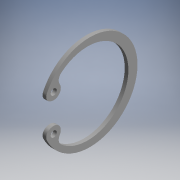
# Autodesk Inventor part: RRING-C-INT-S-30
Saved by Autodesk Inventor 2017.3 (Build 213256000, 256)
## iProperties
Part Number: RRING-C-INT-S-30
Material: Generic
Catalog Web Link: www.cadenas.de
Description: RRING_C_INT-Retaining Rings - C  (Internal)
Vendor: MISUMI
Document SubType Name: Modeling
Designer: partserver
Manufacturer: MISUMI
Mass: 0.253021 g
Surface Area: 6.4299 cm^2
Volume: 0.253021 cm^3
Density: 1 g/cm^3
Appearance: PSOLRGB-192-192-192
Category: PARTsolutions
Company: MISUMI
Title: RRING-C-INT-S-30
Author: Cadenas PARTsolutions
Comments: Retaining Rings - C  (Internal)
PSOL_IDENT_0: {$CADENAS_DATA\23d-libs\misumi\metric\accessories\rring_c_int.prj},181 {VTYP=3D},{NB=RRING-C-INT-S-3
PSOL_IDENT_1: 0},{LINA=RRING-C-INT-S-30},{NN=RRING_C_INT},{DATE=30.10.2020 15:47:10},{GEOMDATE=05.03.2015 00:00:00
PSOL_IDENT_2: },{VERSION=},{LINEID=160},{WBVAR=MAT},{WBNUMERIC=}  {NB=RRING-C-INT-S-30},{LINA=RRING-C-INT-S-30},{K
PSOL_IDENT_3: T=DUMMY},{PN=RRING-C-INT-S-30},{TYPE=RRING-C-INT},{MAT=-S},{HARD=36~44HRC},{NO=30},{DD3=32.1},{DD3TO
PSOL_IDENT_4: L=+0.25/-0.25},{TT=1.20},{TTTOL=+0.06/-0.06},{BB=3.0},{AA=4.7},{DD0=2.0},{DD4=20},{DD1=30},{DD2=31.4
PSOL_IDENT_5: },{DD2TOL=+0.25/0},{MM=1.35},{MMTOL=+0.14/0},{NN=1.5},{A2=12.00}
NB: RRING-C-INT-S-30
NN: 1.5
NT: Retaining Rings - C  (Internal)
NBSYN: $PN.
LINA: RRING-C-INT-S-30
CATALOG: Misumi
PN: RRING-C-INT-S-30
MAT: 304 Stainless Steel-CSP
HARD: 36~44HRC
NO: 30
DD3: 32.1
DD3TOL: +0.25/-0.25
TT: 1.2
TTTOL: +0.06/-0.06
BB: 3
AA: 4.7
DD0: 2
DD4: 20
DD1: 30
DD2: 31.4
DD2TOL: +0.25/0
MM: 1.35
MMTOL: +0.14/0
SUPPLIER: MISUMI
ARTICLENO: RRING-C-INT-S-30
BOMINFO: RRING-C-INT-S-30
CREATOR: CADENAS GmbH
Autodesk Inventor part; units mm, degrees
sketch "Sketch_3" plane through (0, 0, 0) normal (1, 0, 0) x (0, 1, 0)
  arc A0 (-14.2333, -6.626) -> (-14.2333, 6.626) centre (0, 0) ccw
  arc A1 (-14.2333, 6.626) -> (-12.9905, 3.865) centre (-12.4201, 5.7819) ccw
  line L0 (-12.9905, 3.865) -> (-12.5959, 3.7476)
  arc A2 (-12.5959, 3.7476) -> (-9.9259, 7.2342) centre (-11.9257, 6) ccw
  arc A3 (-9.4453, 10.2613) -> (-9.9259, 7.2342) centre (-7.9261, 8.4684) ccw
  arc A4 (-9.4453, -10.2613) -> (-9.4453, 10.2613) centre (-0.75, 0) ccw
  arc A5 (-9.9259, -7.2342) -> (-9.4453, -10.2613) centre (-7.9261, -8.4684) ccw
  arc A6 (-9.9259, -7.2342) -> (-12.5959, -3.7476) centre (-11.9257, -6) ccw
  line L1 (-12.5959, -3.7476) -> (-12.9905, -3.865)
  arc A7 (-12.9905, -3.865) -> (-14.2333, -6.626) centre (-12.4201, -5.7819) ccw
  circle A8 centre (-11.9257, -6) radius 1
  circle A9 centre (-11.9257, 6) radius 1
  constraints: 16 point on circle, 10 centre point, 4 end point
extrude "Extrusion1" add sketch "Sketch_3" along normal mid plane 1.2
ref_plane "rr_XY" through (-0.6, 0, 0) normal (1, 0, 0) x (0, 0, -1)
ref_plane "rr_YZ" through (-0.6, 0, 0) normal (0, 0, -1) x (0, 1, 0)
ref_plane "rr_ZX" through (-0.6, 0, 0) normal (0, 1, 0) x (1, 0, 0)
body "Solid1"
